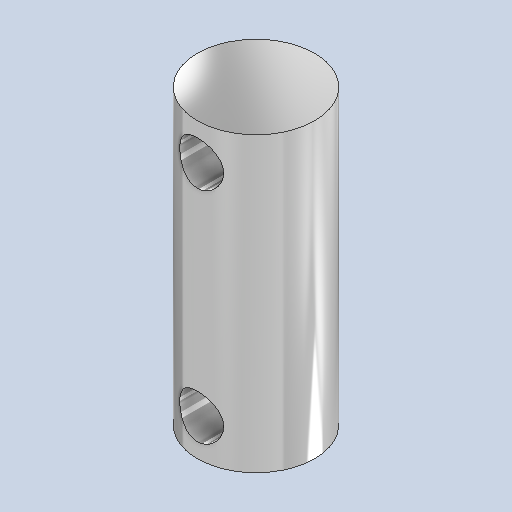
# Autodesk Inventor part: 201 part 22
Saved by Autodesk Inventor 2025.1 (Build 291241000, 241)
## iProperties
Created: 2024-08-01
Part Number: 201 part 22
Material: Aluminum 6061-AHC
Document SubType Name: Modeling
Designer: ffogue
Density: 2.7 g/cm^3
Appearance: Aluminum - Dark
Author: ffogue
Autodesk Inventor part; units mm, degrees
ref_plane "YZ Plane" through (0, 0, 0) normal (1, 0, 0) x (0, 1, 0)
ref_plane "XY Plane" through (0, 0, 0) normal (0, 0, 1) x (1, 0, 0)
sketch "Sketch1" plane through (0, 0, 0) normal (0, 0, 1) x (1, 0, 0)
  circle A0 centre (0, 15) radius 4 projected
  point P0 (0, 0)
extrude "Extrusion1" add sketch "Sketch1" against normal blind 20
ref_plane "Work Plane1" through (0, 19, 0) normal (0, 1, 0) x (-1, 0, 0)
sketch "Sketch2" plane through (0, 19, 0) normal (0, 1, 0) x (-1, 0, 0)
  line L0 (-4, -20) -> (4, -20) projected
  line L1 (4, 0) -> (-4, 0) projected
  point P0 (0, 0)
  point P1 (0, -2.5)
  point P2 (0, -17.5)
  dimension "d3" = 2.5
  dimension "d4" = 2.5
  constraints: 2 vertical alignment
  measures "d3" distance from line of L0 point (0, -17.5)
  measures "d4" distance from line of L1 point (0, -2.5)
hole "Hole1" at (0, 19, -2.5) at (0, 19, -17.5) direction (0, -1, 0) diameter 3 end through all
equation "\"d4\" = d3"
body "Solid1"
